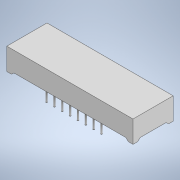
# Autodesk Inventor part: TDCR1050M
Saved by Autodesk Inventor 2020 (Build 240168000, 168)
## iProperties
Created: 2020-11-14
Part Number: TDCR1050M
Material: Generic
Document SubType Name: Modeling
Designer: Admin
Density: 1 g/cm^3
Appearance: Default
Author: Admin
Autodesk Inventor part; units mm, degrees
ref_plane "YZ Plane" through (0, 0, 0) normal (1, 0, 0) x (0, 1, 0)
ref_plane "XZ Plane" through (0, 0, 0) normal (0, 1, 0) x (-1, 0, 0)
ref_plane "XY Plane" through (0, 0, 0) normal (0, 0, 1) x (1, 0, 0)
sketch "Sketch1" plane through (0, 0, 0) normal (0, 0, 1) x (1, 0, 0)
  line L0 (0, 0) -> (40.2, 0)
  line L1 (40.2, 0) -> (40.2, 7)
  line L2 (40.2, 7) -> (0, 7)
  line L3 (0, 7) -> (0, 0)
  constraints: 8 end point, 2 parallel, 1 horizontal, 1 perpendicular
extrude "Extrusion1" add sketch "Sketch1" against normal blind 12.8
sketch "Sketch2" plane through (0, 0, 0) normal (0, 0, 1) x (1, 0, 0)
  line L0 (40.2, 0) -> (0, 0) projected
  line L1 (0, 0) -> (1.2929, 0)
  line L2 (40.2, 7) -> (40.2, 0) projected
  line L3 (40.2, 0) -> (38.9071, 0)
  line L4 (1.5, 0) -> (38.7, 0)
  line L5 (37.7429, 0.75) -> (2.4571, 0.75)
  line L6 (38.5536, 0.1464) -> (38.0964, 0.6036)
  line L7 (1.6464, 0.1464) -> (2.1036, 0.6036)
  arc A0 (2.4571, 0.75) -> (2.1036, 0.6036) centre (2.4571, 0.25) ccw
  arc A1 (1.2929, 0) -> (1.6464, 0.1464) centre (1.2929, 0.5) ccw
  arc A2 (38.0964, 0.6036) -> (37.7429, 0.75) centre (37.7429, 0.25) ccw
  arc A3 (38.5536, 0.1464) -> (38.9071, 0) centre (38.9071, 0.5) ccw
  line L8 (38.9071, 0) -> (1.2929, 0)
  dimension "d2" = 0.5
  constraints: 14 end point, 10 tangent, 8 point on circle, 6 point on line, 4 centre point, 3 equal radius, 1 collinear, 1 horizontal, 1 parallel
  measures "d2" radius of A0
extrude "Extrusion2" cut sketch "Sketch2" against normal through all
sketch "Sketch3" plane through (40.2, 0, 0) normal (1, 0, 0) x (0, 0, -1)
  line L0 (0, 0) -> (12.8, 0) projected
  line L1 (0, 0) -> (1.2929, 0)
  line L2 (12.8, 0) -> (11.5071, 0)
  line L3 (1.5, 0) -> (11.3, 0)
  line L4 (10.3429, 0.75) -> (2.4571, 0.75)
  line L5 (11.1536, 0.1464) -> (10.6964, 0.6036)
  line L6 (1.6464, 0.1464) -> (2.1036, 0.6036)
  arc A0 (2.4571, 0.75) -> (2.1036, 0.6036) centre (2.4571, 0.25) ccw
  arc A1 (1.2929, 0) -> (1.6464, 0.1464) centre (1.2929, 0.5) ccw
  arc A2 (10.6964, 0.6036) -> (10.3429, 0.75) centre (10.3429, 0.25) ccw
  arc A3 (11.1536, 0.1464) -> (11.5071, 0) centre (11.5071, 0.5) ccw
  line L7 (1.2929, 0) -> (11.5071, 0)
  dimension "d5" = 0.5
  constraints: 14 end point, 8 point on circle, 8 tangent, 6 point on line, 4 centre point, 3 equal radius, 1 collinear, 1 horizontal, 1 parallel
  measures "d5" radius of A0
extrude "Extrusion3" cut sketch "Sketch3" against normal through all
sketch "Sketch4" plane through (2.4571, 0.75, 0) normal (0, -1, 0) x (1, 0, 0)
  line L0 (37.7429, -2.4571) -> (37.7429, -10.3429) projected
  line L1 (-2.4571, 0) -> (-2.4571, -12.8) projected
  line L2 (17.6429, -1.32) -> (18.8929, -1.32)
  line L3 (17.6429, -1.32) -> (16.3929, -1.32)
  circle A0 centre (18.8929, -1.32) radius 0.25
  circle A1 centre (21.3929, -1.32) radius 0.25
  circle A2 centre (23.8929, -1.32) radius 0.25
  circle A3 centre (26.3929, -1.32) radius 0.25
  circle A4 centre (16.3929, -1.32) radius 0.25
  circle A5 centre (13.8929, -1.32) radius 0.25
  circle A6 centre (11.3929, -1.32) radius 0.25
  circle A7 centre (8.8929, -1.32) radius 0.25
  circle A8 centre (18.8929, -11.48) radius 0.25
  circle A9 centre (21.3929, -11.48) radius 0.25
  circle A10 centre (23.8929, -11.48) radius 0.25
  circle A11 centre (26.3929, -11.48) radius 0.25
  circle A12 centre (16.3929, -11.48) radius 0.25
  circle A13 centre (13.8929, -11.48) radius 0.25
  circle A14 centre (11.3929, -11.48) radius 0.25
  circle A15 centre (8.8929, -11.48) radius 0.25
  dimension "d10" = 2.5
  dimension "d17" = 2.5
  constraints: 16 centre point, 4 end point, 4 horizontal, 1 coincident, 14 other
  measures "d10" distance of A0.centre A1.centre
  measures "d17" distance of A0.centre A4.centre
extrude "Extrusion4" add sketch "Sketch4" along normal blind 4.25
fillet "Fillet1" radius 0.125 16 edges at (28.6, -3.5, -11.48) (26.1, -3.5, -11.48) (23.6, -3.5, -11.48) (21.1, -3.5, -11.48) (18.6, -3.5, -11.48) (16.1, -3.5, -11.48) (13.6, -3.5, -11.48) (11.1, -3.5, -11.48) (11.1, -3.5, -1.32) (13.6, -3.5, -1.32) (16.1, -3.5, -1.32) (18.6, -3.5, -1.32) (21.1, -3.5, -1.32) (23.6, -3.5, -1.32) (26.1, -3.5, -1.32) (28.6, -3.5, -1.32)
body "Solid1"
